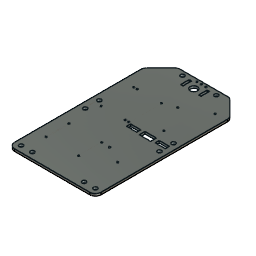
base_piso_2_electronica (Autodesk Fusion 360 design; units mm, degrees)
Autodesk Fusion 360 part; units mm, degrees
note: some values were not read from the file. Chosen so that the rebuilt part matches the saved one: which face or edge a step refers to. Set by a fixed rule: which sketch regions a step uses.
imported_body "Operación base derivada4" makes body 1
imported_body "Operación base derivada5" makes body 2
imported_body "Operación base derivada6" makes body 3
imported_body "Operación base derivada7" makes body 4
imported_body "Operación base derivada8" makes body 5
sketch "Boceto1" plane through (0, 0, 0) normal (0, 0, 1) x (1, 0, 0)
  line L0 (-77.0741, -35.0015) -> (-77.0741, -116.763)
  line L1 (-0.0741, 152.5) -> (-0.0741, -130) construction
  line L2 (-80, 72.5) -> (80.1608, 72.5) construction
  arc A0 (-78.7959, 73.6379) -> (-79.0142, 70.8179) centre (-77.4951, 72.1188) ccw
  line L3 (-120, 0) -> (120, 0) construction
  arc A1 (78.866, 70.8179) -> (78.6478, 73.6379) centre (77.3469, 72.1188) ccw
  line L4 (-74.1452, 115.3418) -> (-48.5931, 140.8939)
  line L5 (-83.6742, 105.8127) -> (-54.7157, 105.8127) construction
  line L6 (-77.0741, 32.4265) -> (-77.0741, -35.0015)
  line L7 (66.9259, 7.737) -> (48.9259, 7.737)
  line L8 (48.9259, 7.737) -> (48.9259, 14.737)
  line L9 (48.9259, 14.737) -> (66.9259, 14.737)
  line L10 (66.9259, 14.737) -> (66.9259, 7.737)
  line L11 (66.9259, 7.737) -> (48.9259, 14.737) construction
  line L12 (48.9259, 7.737) -> (66.9259, 14.737) construction
  line L13 (42.4259, 5.9107) -> (42.4259, 15.9107)
  line L14 (42.4259, 15.9107) -> (22.4259, 15.9107)
  line L15 (22.4259, 15.9107) -> (22.4259, 5.9107)
  line L16 (22.4259, 5.9107) -> (42.4259, 5.9107)
  arc A2 (-42.9362, 143.237) -> (-48.5931, 140.8939) centre (-42.9362, 135.237) ccw
  circle A3 centre (-30.0741, 135.237) radius 3.5
  circle A4 centre (-66.0741, 23.237) radius 3.5
  circle A5 centre (-66.0741, -115.763) radius 3.5
  circle A6 centre (29.9259, 135.237) radius 3.5
  circle A7 centre (65.9259, 23.237) radius 3.5
  line L17 (-77.0741, 32.4265) -> (-77.0741, 108.2707)
  arc A8 (-74.1452, 115.3418) -> (-77.0741, 108.2707) centre (-67.0741, 108.2707) ccw
  arc A9 (48.4449, 140.8939) -> (42.788, 143.237) centre (42.788, 135.237) ccw
  line L18 (-42.9362, 143.237) -> (42.788, 143.237)
  arc A10 (76.9259, 108.2707) -> (73.997, 115.3418) centre (66.9259, 108.2707) ccw
  line L19 (73.997, 115.3418) -> (48.4449, 140.8939)
  line L20 (76.9259, 32.4265) -> (76.9259, 108.2707)
  line L21 (76.9259, 32.4265) -> (76.9259, -35.0015)
  line L22 (76.9259, -35.0015) -> (76.9259, -116.763)
  line L23 (-67.0741, -126.763) -> (66.9259, -126.763)
  arc A11 (66.9259, -126.763) -> (76.9259, -116.763) centre (66.9259, -116.763) ccw
  arc A12 (-77.0741, -116.763) -> (-67.0741, -126.763) centre (-67.0741, -116.763) ccw
  circle A13 centre (65.9259, -115.763) radius 3.5
  circle A14 centre (-46.0741, -115.763) radius 3.5
  circle A15 centre (45.9259, -115.763) radius 3.5
  circle A16 centre (-66.0741, -1.763) radius 3.5
  circle A17 centre (65.9259, -1.763) radius 3.5
  circle A18 centre (-0.0741, 125.237) radius 6.5
  circle A19 centre (-8.0741, 138.737) radius 1.5
  circle A20 centre (7.9259, 138.737) radius 1.5221
  circle A21 centre (-0.0741, 138.737) radius 1.5
  line L24 (10.458, 172.2774) -> (-10.542, 172.2774)
  circle A22 centre (7.958, 167.7774) radius 1.5
  arc A23 (12.458, 170.2774) -> (10.458, 172.2774) centre (10.458, 170.2774) ccw
  line L25 (12.458, 163.2774) -> (12.458, 170.2774)
  arc A24 (-10.542, 172.2774) -> (-12.542, 170.2774) centre (-10.542, 170.2774) ccw
  circle A25 centre (-8.042, 167.7774) radius 1.5
  circle A26 centre (-0.042, 167.7774) radius 1.5
  line L26 (-12.542, 163.2774) -> (12.458, 163.2774)
  line L27 (-12.542, 170.2774) -> (-12.542, 163.2774)
  line L28 (-18.0741, 135) -> (-14.0741, 135)
  line L29 (-14.0741, 135) -> (-14.0741, 120)
  line L30 (-14.0741, 120) -> (-18.0741, 120)
  line L31 (-18.0741, 120) -> (-18.0741, 135)
  circle A27 centre (-8.0741, 138.737) radius 1.5221
  line L32 (13.9259, 120) -> (17.9259, 120)
  line L33 (13.9259, 135) -> (13.9259, 120)
  line L34 (17.9259, 120) -> (17.9259, 135)
  line L35 (17.9259, 135) -> (13.9259, 135)
  line L36 (-2.0741, 7.737) -> (15.9259, 14.737) construction
  line L37 (15.9259, 7.737) -> (-2.0741, 7.737)
  line L38 (15.9259, 7.737) -> (-2.0741, 14.737) construction
  line L39 (-2.0741, 14.737) -> (15.9259, 14.737)
  line L40 (15.9259, 14.737) -> (15.9259, 7.737)
  line L41 (-2.0741, 7.737) -> (-2.0741, 14.737)
  circle A28 centre (-55.6911, 74.1463) radius 1.3645
  circle A29 centre (-66.1112, 23.2764) radius 3.5
  circle A30 centre (-55.6911, 16.0608) radius 1.3645
  circle A31 centre (-6.6911, 16.0608) radius 1.3645
  circle A32 centre (-6.6911, 74.1463) radius 1.3645
  circle A33 centre (-49.6422, 74.1791) radius 1.5
  circle A34 centre (-12.8902, 16.4094) radius 1.5
  circle A35 centre (-66.0966, -1.7742) radius 3.5
  circle A36 centre (-57.2943, -39.2936) radius 1.5
  circle A37 centre (15.2178, -39.6475) radius 1.75
  circle A38 centre (-66.0966, -1.7742) radius 3.5
  circle A39 centre (0.7057, -39.2936) radius 1.5
  circle A40 centre (-66.0966, -1.7742) radius 3.5
  circle A41 centre (-57.2943, -80.2936) radius 1.5
  circle A42 centre (45.2178, -55.6475) radius 1.5
  circle A43 centre (0.7057, -80.2936) radius 1.5
  line L42 (48.8659, 14.6587) -> (66.9253, 14.7383)
  line L43 (66.9253, 14.7383) -> (66.8659, 7.6587)
  circle A44 centre (37.9871, 33.8995) radius 1.5
  circle A45 centre (37.9871, 33.8995) radius 1.5
  circle A46 centre (57.6671, 105.4795) radius 1.5
  circle A47 centre (57.6671, 105.4795) radius 1.5
  circle A48 centre (14.7871, 81.9795) radius 1.5
  circle A49 centre (14.7871, 81.9795) radius 1.5
  circle A50 centre (-9.1129, 93.5031) radius 0.175
  line L44 (48.8659, 7.6587) -> (48.8659, 14.6587)
  line L45 (66.8659, 7.6587) -> (48.8659, 7.6587)
  point P0 (-45.8598, 143.6271)
  point P1 (47.4167, 143.5198)
  point P2 (-82.9449, -126.3729)
  point P3 (57.9259, 11.237)
  point P4 (6.9259, 11.237)
  point P5 (-1.242, 6.4413)
  dimension "d14" = 2
  dimension "d54" = 45
  dimension "d72" = 18
  dimension "d73" = 7
  dimension "d109" = 8
  dimension "d116" = 7
  dimension "d118" = 30
  dimension "d119" = 7
  dimension "d120" = 11
  dimension "d122" = 7
  dimension "d128" = 20
  dimension "d130" = 10
  dimension "d132" = 11
  dimension "d137" = 10
  dimension "d140" = 77
  dimension "d141" = 10
  dimension "d142" = 10
  dimension "d143" = 8
  dimension "d144" = 11
  dimension "d145" = 150
  dimension "d146" = 270
  dimension "d147" = 7
  dimension "d148" = 20
  dimension "d149" = 7
  dimension "d154" = 25
  dimension "d155" = 11
  dimension "d156" = 13
  dimension "d157" = 18
  dimension "d158" = 8
  dimension "d159" = 4.5
  dimension "d160" = 8
  dimension "d161" = 8
  dimension "d162" = 8
  dimension "d163" = 4.5
  dimension "d164" = 4
  dimension "d165" = 15
  dimension "d166" = 14
  dimension "d167" = 10
  dimension "d168" = 18
  dimension "d169" = 7
  dimension "d170" = 132
  dimension "d171" = 132
  dimension "d175" = 6.5
  dimension "d176" = 6.5
  constraint vertical L0
  constraint symmetric L1 A0.start A1.end
  constraint symmetric L1 A0.end A1.start
  constraint symmetric L1 A0 A1
  constraint horizontal L5
  constraint parallel L0 L6
  constraint horizontal L7
  constraint perpendicular L7 L8
  constraint parallel L7 L9
  constraint parallel L8 L10
  constraint coincident L11 P3
  constraint coincident L12 P3
  constraint perpendicular L13 L14
  constraint parallel L13 L15
  constraint parallel L14 L16
  constraint coincident L5.start L4
  constraint coincident P0 L4
  constraint tangent L4 A2
  constraint symmetric L1 A3 A6
  constraint symmetric L1 A4 A7
  constraint vertical L17
  constraint tangent L4 A8
  constraint tangent L17 A8
  constraint symmetric L1 A2.start A9.end
  constraint symmetric L1 L4.end A9.start
  constraint symmetric L1 A2 A9
  constraint tangent A9 L18
  constraint symmetric L0.start L1 L21.end
  constraint symmetric L1 L6.start L20.start
  constraint symmetric L1 L4.start A10.end
  constraint symmetric L1 L17.end A10.start
  constraint symmetric L1 A8 A10
  constraint tangent L22 A11
  constraint tangent L23 A11
  constraint tangent L0 A12
  constraint tangent L23 A12
  constraint symmetric L1 A5 A13
  constraint symmetric L1 A14 A15
  constraint symmetric L1 A16 A17
  constraint coincident L1 A18.centre
  constraint coincident L1 A21.centre
  constraint horizontal L28
  constraint vertical L29
  constraint horizontal L30
  constraint vertical L31
  constraint symmetric L1 A20 A27
  constraint symmetric L1 L28.start L34.end
  constraint symmetric L1 L28.end L33.start
  constraint symmetric L1 L29.end L32.start
  constraint symmetric L1 L30.end L32.end
  constraint horizontal L37
  constraint perpendicular L37 L41
  constraint parallel L37 L39
  constraint parallel L40 L41
  constraint coincident P4 L38
  constraint coincident P4 L36
  measures "d14" radius of A0
  measures "d54" angle of L4 L5
  measures "d72" distance of L8.end L9.end
  measures "d73" distance of L7.end L8.end
  measures "d109" radius of A2
  measures "d116" diameter of A3
  measures "d118" distance of L1 A3.centre
  measures "d119" diameter of A4
  measures "d120" distance of L6 A4.centre
  measures "d122" diameter of A5
  measures "d128" distance of L13.end L14.end
  measures "d130" distance of L14.end L15.end
  measures "d132" distance of L0 A5.centre
  measures "d137" radius of A8
  measures "d140" distance of L0 L1
  measures "d141" radius of A11
  measures "d142" radius of A12
  measures "d143" distance of A3.centre L18
  measures "d144" distance of A5.centre L23
  measures "d145" distance of A4.centre L23
  measures "d146" vertical distance of A2.start L23.start
  measures "d147" diameter of A14
  measures "d148" distance of A5.centre A14.centre
  measures "d149" diameter of A16
  measures "d154" vertical distance of A4.centre A16.centre
  measures "d155" distance of L6 A16.centre
  measures "d156" diameter of A18
  measures "d157" distance of L18 A18.centre
  measures "d158" distance of A26.centre A22.centre
  measures "d159" distance of A26.centre L24
  measures "d160" distance of A21.centre A20.centre
  measures "d161" distance of A21.centre A19.centre
  measures "d162" distance of A26.centre A25.centre
  measures "d163" distance of L18 A21.centre
  measures "d164" distance of L28.start L28.end
  measures "d165" distance of L28.start L30.end
  measures "d166" distance of L1 L29
  measures "d167" distance of L10 L21
  measures "d168" distance of L38.end L36.end
  measures "d169" distance of L38.end L36.start
  measures "d170" vertical distance of P3 A9.end
  measures "d171" distance of L18 P4
  measures "d175" distance of L8 L13
  measures "d176" distance of L15 L40
extrude "Extruir7" add sketch "Boceto1" along normal blind 4 separate body contours L0 L4 L6 A2 L17 A8 A9 L18 A10 L19 L20 L21 L22 L23 A11 A12 | L7 L8 L42 L43 L44 L45 | A4 A29 | A16 A35 A38 A40 | A50 picked at (-68.4835, 25.7916) picked at (-69.1741, -3.405) makes body 6
sketch "Boceto5" plane through (0, 0, 4) normal (0, 0, 1) x (-1, 0, 0)
  line L0 (-13.9259, -135) -> (-17.9259, -135)
  line L1 (-17.9259, -135) -> (-17.9259, -120)
  line L2 (-17.9259, -120) -> (-13.9259, -120)
  line L3 (-13.9259, -120) -> (-13.9259, -135)
  circle A0 centre (-7.9259, -138.737) radius 1.5221
  circle A1 centre (-65.9259, 115.763) radius 3.5
  circle A2 centre (6.6911, -16.0608) radius 1.3645
  circle A3 centre (30.0741, -135.237) radius 3.5
  circle A4 centre (-0.7057, 39.2936) radius 1.5
  circle A5 centre (66.0741, 1.763) radius 3.5
  circle A6 centre (8.0741, -138.737) radius 1.5221
  circle A7 centre (12.8902, -16.4094) radius 1.5
  circle A8 centre (57.2943, 39.2936) radius 1.5
  circle A9 centre (66.0741, 115.763) radius 3.5
  circle A10 centre (55.6911, -16.0608) radius 1.3645
  circle A11 centre (-0.7057, 80.2936) radius 1.5
  circle A12 centre (6.6911, -74.1463) radius 1.3645
  circle A13 centre (55.6911, -74.1463) radius 1.3645
  circle A14 centre (66.0741, -23.237) radius 3.5
  circle A15 centre (-65.9259, 1.763) radius 3.5
  circle A16 centre (-15.2178, 39.6475) radius 1.75
  line L4 (-42.4259, -5.9107) -> (-22.4259, -5.9107)
  line L5 (-22.4259, -5.9107) -> (-22.4259, -15.9107)
  line L6 (-22.4259, -15.9107) -> (-42.4259, -15.9107)
  line L7 (-42.4259, -15.9107) -> (-42.4259, -5.9107)
  circle A17 centre (0.0741, -125.237) radius 6.5
  circle A18 centre (-45.2178, 55.6475) radius 1.5
  circle A19 centre (46.0741, 115.763) radius 3.5
  circle A20 centre (0.0741, -138.737) radius 1.5
  circle A21 centre (57.2943, 80.2936) radius 1.5
  circle A22 centre (-45.9259, 115.763) radius 3.5
  circle A23 centre (49.6422, -74.1791) radius 1.5
  circle A24 centre (-29.9259, -135.237) radius 3.5
  circle A25 centre (-65.9259, -23.237) radius 3.5
  line L8 (14.0741, -120) -> (18.0741, -120)
  line L9 (18.0741, -120) -> (18.0741, -135)
  line L10 (18.0741, -135) -> (14.0741, -135)
  line L11 (14.0741, -135) -> (14.0741, -120)
  line L12 (-48.9259, -14.737) -> (-66.9259, -14.737)
  line L13 (-66.9259, -14.737) -> (-66.9259, -7.737)
  line L14 (-66.9259, -7.737) -> (-48.9259, -7.737)
  line L15 (-48.9259, -7.737) -> (-48.9259, -14.737)
  line L16 (-15.9259, -7.737) -> (2.0741, -7.737)
  line L17 (2.0741, -7.737) -> (2.0741, -14.737)
  line L18 (2.0741, -14.737) -> (-15.9259, -14.737)
  line L19 (-15.9259, -14.737) -> (-15.9259, -7.737)
  line L20 (77.0741, -108.2707) -> (77.0741, 116.763)
  arc A26 (77.0741, 116.763) -> (67.0741, 126.763) centre (67.0741, 116.763) ccw
  line L21 (67.0741, 126.763) -> (-66.9259, 126.763)
  arc A27 (-66.9259, 126.763) -> (-76.9259, 116.763) centre (-66.9259, 116.763) ccw
  line L22 (-76.9259, 116.763) -> (-76.9259, -108.2707)
  arc A28 (-76.9259, -108.2707) -> (-73.997, -115.3418) centre (-66.9259, -108.2707) ccw
  line L23 (-73.997, -115.3418) -> (-48.4449, -140.8939)
  arc A29 (-48.4449, -140.8939) -> (-42.788, -143.237) centre (-42.788, -135.237) ccw
  line L24 (-42.788, -143.237) -> (42.9362, -143.237)
  arc A30 (42.9362, -143.237) -> (48.5931, -140.8939) centre (42.9362, -135.237) ccw
  line L25 (48.5931, -140.8939) -> (74.1452, -115.3418)
  arc A31 (74.1452, -115.3418) -> (77.0741, -108.2707) centre (67.0741, -108.2707) ccw
  circle A32 centre (-57.6671, -105.4795) radius 1.5
  circle A33 centre (-14.7871, -81.9795) radius 1.5
  circle A34 centre (-37.9871, -33.8995) radius 1.5
sketch "Boceto6" plane through (0, 0, 4) normal (0, 0, 1) x (-1, 0, 0)
  circle A0 centre (66.0741, 1.763) radius 3.5
  circle A1 centre (66.0741, -23.237) radius 3.5
  line L0 (-48.9259, -14.737) -> (-66.9259, -14.737)
  line L1 (-66.9259, -14.737) -> (-66.9259, -7.737)
  line L2 (-66.9259, -7.737) -> (-48.9259, -7.737)
  line L3 (-48.9259, -7.737) -> (-48.9259, -14.737)
  circle A2 centre (46.0741, 115.763) radius 3.5
  circle A3 centre (30.0741, -135.237) radius 3.5
  circle A4 centre (-45.9259, 115.763) radius 3.5
  line L4 (-42.4259, -5.9107) -> (-22.4259, -5.9107)
  line L5 (-22.4259, -5.9107) -> (-22.4259, -15.9107)
  line L6 (-22.4259, -15.9107) -> (-42.4259, -15.9107)
  line L7 (-42.4259, -15.9107) -> (-42.4259, -5.9107)
  line L8 (-13.9259, -135) -> (-17.9259, -135)
  line L9 (-17.9259, -135) -> (-17.9259, -120)
  line L10 (-17.9259, -120) -> (-13.9259, -120)
  line L11 (-13.9259, -120) -> (-13.9259, -135)
  circle A5 centre (0.0741, -125.237) radius 6.5
  circle A6 centre (55.6911, -74.1463) radius 1.3645
  circle A7 centre (-65.9259, -23.237) radius 3.5
  circle A8 centre (-7.9259, -138.737) radius 1.5221
  line L12 (-15.9259, -7.737) -> (2.0741, -7.737)
  line L13 (2.0741, -7.737) -> (2.0741, -14.737)
  line L14 (2.0741, -14.737) -> (-15.9259, -14.737)
  line L15 (-15.9259, -14.737) -> (-15.9259, -7.737)
  circle A9 centre (6.6911, -74.1463) radius 1.3645
  circle A10 centre (8.0741, -138.737) radius 1.5221
  circle A11 centre (49.6422, -74.1791) radius 1.5
  circle A12 centre (12.8902, -16.4094) radius 1.5
  circle A13 centre (55.6911, -16.0608) radius 1.3645
  circle A14 centre (-29.9259, -135.237) radius 3.5
  circle A15 centre (-65.9259, 1.763) radius 3.5
  circle A16 centre (-65.9259, 115.763) radius 3.5
  circle A17 centre (66.0741, 115.763) radius 3.5
  circle A18 centre (57.2943, 80.2936) radius 1.5
  circle A19 centre (-57.6671, -105.4795) radius 1.5
  circle A20 centre (-14.7871, -81.9795) radius 1.5
  circle A21 centre (-37.9871, -33.8995) radius 1.5
  circle A22 centre (-0.7057, 39.2936) radius 1.5
  circle A23 centre (-15.2178, 39.6475) radius 1.75
  circle A24 centre (57.2943, 39.2936) radius 1.5
  circle A25 centre (6.6911, -16.0608) radius 1.3645
  line L16 (14.0741, -120) -> (18.0741, -120)
  line L17 (18.0741, -120) -> (18.0741, -135)
  line L18 (18.0741, -135) -> (14.0741, -135)
  line L19 (14.0741, -135) -> (14.0741, -120)
  circle A26 centre (-45.2178, 55.6475) radius 1.5
  circle A27 centre (-0.7057, 80.2936) radius 1.5
  circle A28 centre (0.0741, -138.737) radius 1.5
  line L20 (77.0741, -108.2707) -> (77.0741, 116.763)
  arc A29 (77.0741, 116.763) -> (67.0741, 126.763) centre (67.0741, 116.763) ccw
  line L21 (67.0741, 126.763) -> (-66.9259, 126.763)
  arc A30 (-66.9259, 126.763) -> (-76.9259, 116.763) centre (-66.9259, 116.763) ccw
  line L22 (-76.9259, 116.763) -> (-76.9259, -108.2707)
  arc A31 (-76.9259, -108.2707) -> (-73.997, -115.3418) centre (-66.9259, -108.2707) ccw
  line L23 (-73.997, -115.3418) -> (-48.4449, -140.8939)
  arc A32 (-48.4449, -140.8939) -> (-42.788, -143.237) centre (-42.788, -135.237) ccw
  line L24 (-42.788, -143.237) -> (42.9362, -143.237)
  arc A33 (42.9362, -143.237) -> (48.5931, -140.8939) centre (42.9362, -135.237) ccw
  line L25 (48.5931, -140.8939) -> (74.1452, -115.3418)
  arc A34 (74.1452, -115.3418) -> (77.0741, -108.2707) centre (67.0741, -108.2707) ccw
hidden bodies 1 2 3 4 5
named bodies: "Cuerpo1 (Contexto3)", "Cuerpo1 (1) (Contexto3)", "Cuerpo1 (2) (Contexto3)", "Cuerpo1 (3) (Contexto3)", "Cuerpo1 (4) (Contexto3)"
